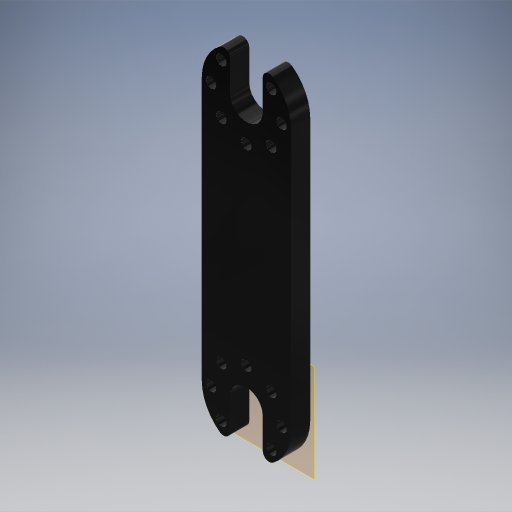
# Autodesk Inventor part: leg_ver2_new
Saved by Autodesk Inventor 2024 (Build 280153000, 153)
## iProperties
Created: 2024-09-04
Part Number: leg_ver2_new
Material: PMMA 플라스틱
Document SubType Name: Modeling
Designer: msi
Density: 1.188 g/cm^3
Appearance: 매끄러움 - 검은색
Author: msi
Autodesk Inventor part; units mm, degrees
ref_plane "YZ Plane" through (0, 0, 0) normal (1, 0, 0) x (0, 1, 0)
ref_plane "XZ Plane" through (0, 0, 0) normal (0, 1, 0) x (-1, 0, 0)
ref_plane "XY Plane" through (0, 0, 0) normal (0, 0, 1) x (1, 0, 0)
ref_plane "작업 평면1" through (0, 0, 0) normal (0, 0, 1) x (1, 0, 0)
sketch "스케치1" plane through (0, 0, 0) normal (0, 0, 1) x (1, 0, 0)
  circle A0 centre (-7.7782, -7.7782) radius 1.55 projected
  circle A1 centre (7.7782, -7.7782) radius 1.55 projected
  circle A2 centre (7.7782, 7.7782) radius 1.55 projected
  circle A3 centre (-7.7782, 7.7782) radius 1.55 projected
  circle A4 centre (0, 0) radius 5 projected
  circle A5 centre (0, 11) radius 1.55 projected
  circle A6 centre (11, 0) radius 1.55 projected
  circle A7 centre (0, -11) radius 1.55 projected
  circle A8 centre (-11, 0) radius 1.55 projected
  circle A9 centre (0, 0) radius 5.1
  line L0 (-13.9, 0) -> (13.9, 0)
  line L1 (13.9, 0) -> (13.9, 13.9)
  line L2 (13.9, 13.9) -> (-13.9, 13.9)
  line L3 (-13.9, 13.9) -> (-13.9, 0)
  line L4 (-5.1, 0) -> (-5.1, -12.9306)
  line L5 (5.1, 0) -> (5.1, -12.9306)
  circle A10 centre (-7.7782, 7.7782) radius 1.6
  circle A11 centre (-11, 0) radius 1.6
  circle A12 centre (-7.7782, -7.7782) radius 1.6
  circle A13 centre (0, -11) radius 1.6
  circle A14 centre (7.7782, -7.7782) radius 1.6
  circle A15 centre (11, 0) radius 1.6
  circle A16 centre (7.7782, 7.7782) radius 1.6
  circle A17 centre (0, 11) radius 1.6
  line L6 (-13.9, 13.9) -> (13.9, 13.9)
  circle A18 centre (-7.7782, -7.7782) radius 1.55 projected
  circle A19 centre (7.7782, -7.7782) radius 1.55 projected
  circle A20 centre (7.7782, 7.7782) radius 1.55 projected
  circle A21 centre (-7.7782, 7.7782) radius 1.55 projected
  circle A22 centre (0, 0) radius 5 projected
  circle A23 centre (0, 0) radius 13.9 projected
  circle A24 centre (0, 11) radius 1.55 projected
  circle A25 centre (11, 0) radius 1.55 projected
  circle A26 centre (0, -11) radius 1.55 projected
  circle A27 centre (-11, 0) radius 1.55 projected
  circle A28 centre (0, 0) radius 13.9
  line L7 (-13.9, 13.9) -> (13.9, 13.9)
  line L8 (13.9, 13.9) -> (13.9, 40.9)
  line L9 (13.9, 40.9) -> (-13.9, 40.9)
  line L10 (-13.9, 40.9) -> (-13.9, 13.9)
  dimension "d0" = 0.1
  dimension "d1" = 3.2
  dimension "d4" = 360
  dimension "d10" = 27
  dimension "d16" = 13.9
  constraints: 22 end point, 10 centre point, 5 parallel, 3 horizontal, 3 perpendicular, 2 coincident, 2 point on circle, 2 point on line, 2 tangent, 1 concentric, 17 other
  measures "d0" radial gap between concentric circles of A4 A9
  measures "d1" diameter of A10
  measures "d10" distance of L8.end L7.end
  measures "d16" distance between parallel lines of L0 L2
extrude "돌출4" add sketch "스케치1" along normal blind 6 contours A9 L0 A11 A23 A15 | L0 A15 A23 L5 | L4 A23 L0 A11 | A23 L2 L1 | L3 L2 A23 | L2 L10 L9 L8
mirror "미러4" about plane through (13.9, 40.9, 0) normal (0, 1, 0)
fillet "모깎기3" radius 2 4 edges at (5.1, 94.7306, 3) (-5.1, 94.7306, 3) (5.1, -12.9306, 3) (-5.1, -12.9306, 3)
